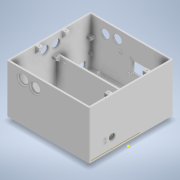
# Autodesk Inventor part: Base
Saved by Autodesk Inventor 2022.2 (Build 262287000, 287)
## iProperties
Created: 2022-01-15
Part Number: Base
Material: Generic
Document SubType Name: Modeling
Designer: siwat
Density: 1 g/cm^3
Appearance: Default
Mass: 201.568 g
Surface Area: 1377.7 cm^2
Volume: 201.568 cm^3
Author: siwat
Autodesk Inventor part; units mm, degrees
ref_plane "YZ Plane" through (0, 0, 0) normal (1, 0, 0) x (0, 1, 0)
ref_plane "XZ Plane" through (0, 0, 0) normal (0, 1, 0) x (-1, 0, 0)
ref_plane "XY Plane" through (0, 0, 0) normal (0, 0, 1) x (1, 0, 0)
ref_plane "Work Plane1" through (31.5112, 10.0003, 59.575) normal (-0.0015858, -0.9999987, 0.0000018) x (-0.0011293, 0, -0.9999994)
sketch "Sketch1" plane through (31.5112, 10.0003, 59.575) normal (-0.0015858, -0.9999987, 0.0000018) x (-0.0011293, 0, -0.9999994)
  line L0 (-4.5224, 4.5326) -> (134.4396, 4.5326)
  line L1 (134.4396, 4.5326) -> (134.4396, -131.8992)
  line L2 (134.4396, -131.8992) -> (-4.5224, -131.8992)
  line L3 (-4.5224, -131.8992) -> (-4.5224, 4.5326)
  line L4 (-7.5224, 7.5326) -> (137.4396, 7.5326)
  line L5 (137.4396, 7.5326) -> (137.4396, -134.8992)
  line L6 (137.4396, -134.8992) -> (-7.5224, -134.8992)
  line L7 (-7.5224, -134.8992) -> (-7.5224, 7.5326)
  point P0 (59.6106, -31.428)
  dimension "d0" = 138.9621
  dimension "d1" = 136.4319
  dimension "d2" = 74.8291
  dimension "d3" = 35.9607
  dimension "d4" = 3
  dimension "d5" = 3
  dimension "d6" = 3
  dimension "d7" = 3
  constraints: 16 end point, 4 parallel, 2 horizontal, 2 perpendicular
  measures "d0" distance between parallel lines of L1 L3
  measures "d1" distance between parallel lines of L0 L2
  measures "d2" distance from line of point (59.611, -31.428) L1
  measures "d3" distance from line of point (59.611, -31.428) L0
  measures "d4" distance between parallel lines of L0 L4
  measures "d5" distance between parallel lines of L3 L7
  measures "d6" distance between parallel lines of L5 L1
  measures "d7" distance between parallel lines of L6 L2
extrude "Extrusion1" add sketch "Sketch1" against normal blind 80
sketch "Sketch2" plane through (31.5112, 10.0003, 59.575) normal (-0.0015858, -0.9999987, 0.0000018) x (0.9999981, -0.0015858, -0.0011293)
  line L0 (-134.8992, -137.4396) -> (7.5326, -137.4396) projected
  line L1 (7.5326, 7.5224) -> (-134.8992, 7.5224) projected
  line L2 (7.5326, -137.4396) -> (-134.8992, -137.4396)
  line L3 (-134.8992, -137.4396) -> (-134.8992, 7.5224)
  line L4 (-134.8992, 7.5224) -> (7.5326, 7.5224)
  line L5 (7.5326, 7.5224) -> (7.5326, -137.4396)
  point P0 (-31.428, -59.6106)
  point P1 (-134.8992, -137.4396)
  point P2 (7.5326, 7.5224)
  constraints: 8 end point, 2 parallel, 1 horizontal, 1 perpendicular
extrude "Extrusion2" add sketch "Sketch2" along normal blind 3
sketch "Sketch3" plane through (31.5112, 10.0003, 59.575) normal (0.0015858, 0.9999987, -0.0000018) x (0.9999981, -0.0015858, -0.0011293)
  circle A0 centre (-112.8782, 129.2967) radius 1.9965
  circle A1 centre (-112.8782, 129.2967) radius 1
  circle A2 centre (-114.2274, 81.024) radius 1.9965
  circle A3 centre (-114.2274, 81.024) radius 1
  circle A4 centre (-62.1401, 86.0453) radius 1.9965
  circle A5 centre (-62.1401, 86.0453) radius 1
  circle A6 centre (-62.0938, 113.9832) radius 1.9965
  circle A7 centre (-62.0938, 113.9832) radius 1
  circle A8 centre (-37.9957, 129.2347) radius 1.9965
  circle A9 centre (-37.9957, 129.2347) radius 1
  circle A10 centre (-31.6312, 80.9446) radius 1.9965
  circle A11 centre (-31.6312, 80.9446) radius 1
  circle A12 centre (-6.6551, 121.5212) radius 2.3058
  circle A13 centre (-6.6551, 121.5212) radius 1
  circle A14 centre (-22.9352, 91.3493) radius 2.3058
  circle A15 centre (-22.9352, 91.3493) radius 1
  circle A16 centre (-129.08, 0.6108) radius 2.6932
  circle A17 centre (-129.08, 0.6108) radius 1
  circle A18 centre (-24.0772, 69.1234) radius 2.8442
  circle A19 centre (-24.0772, 69.1234) radius 1
  point P0 (-31.428, 59.6106)
  dimension "d12" = 2
  dimension "d13" = 2
  dimension "d14" = 2
  dimension "d15" = 2
  dimension "d16" = 2
  dimension "d17" = 2
  dimension "d18" = 2
  dimension "d19" = 2
  dimension "d28" = 2
  dimension "d29" = 2
  constraints: 20 centre point, 10 coincident
  measures "d12" diameter of A1
  measures "d13" diameter of A3
  measures "d14" diameter of A5
  measures "d15" diameter of A7
  measures "d16" diameter of A9
  measures "d17" diameter of A11
  measures "d18" diameter of A13
  measures "d19" diameter of A15
  measures "d28" diameter of A17
  measures "d29" diameter of A19
extrude "Extrusion3" add sketch "Sketch3" along normal blind 5
sketch "Sketch4" plane through (31.5112, 10.0003, 59.575) normal (0.0015858, 0.9999987, -0.0000018) x (0.9999981, -0.0015858, -0.0011293)
  line L0 (4.5326, 134.4396) -> (4.5326, -4.5224) projected
  line L1 (-131.8992, 134.4396) -> (-131.8992, -4.5224) projected
  line L2 (4.5326, 74.8611) -> (-131.8992, 74.8611)
  line L3 (-131.8992, 74.8611) -> (-131.8992, 77.8611)
  line L4 (-131.8992, 77.8611) -> (4.5326, 77.8611)
  line L5 (4.5326, 77.8611) -> (4.5326, 74.8611)
  point P0 (-31.428, 59.6106)
  point P1 (4.5326, 77.8611)
  point P2 (-131.8992, 74.8611)
  dimension "d22" = 3
  constraints: 8 end point, 2 parallel, 2 point on line, 1 horizontal, 1 perpendicular
  measures "d22" distance between parallel lines of L4 L2
extrude "Extrusion4" add sketch "Sketch4" along normal blind 50
sketch "Sketch5" plane through (35.9559, 9.9931, -18.2911) normal (-0.0011293, 0, -0.9999994) x (-0.9999981, 0.0015858, 0.0011293)
  circle A0 centre (12.779, 19.6609) radius 10
  point P0 (35.9607, -10.0501)
  dimension "d25" = 20
  constraints: 1 centre point
  measures "d25" diameter of A0
extrude "Extrusion5" cut sketch "Sketch5" against normal up to surface (3 mm away)
sketch "Sketch7" plane through (-100.5396, 10.2094, -74.7156) normal (0.9999981, -0.0015858, -0.0011293) x (-0.0011293, 0, -0.9999994)
  line L0 (0, 0) -> (0, 80) projected
  line L1 (0, 24.9377) -> (-4, 24.9377)
  line L2 (-4, 24.9377) -> (-4, 20.9377)
  line L3 (-4, 20.9377) -> (0, 20.9377)
  line L4 (0, 20.9377) -> (0, 24.9377)
  line L5 (-4, 24.9377) -> (-56.5786, 24.9377)
  line L6 (-56.5786, 50) -> (-56.5786, 0) projected
  line L7 (-4, 20.9377) -> (-56.5786, 20.9377)
  line L8 (-52.5786, 24.9377) -> (-52.5786, 20.9377)
  line L9 (-56.5786, 0) -> (-56.5786, 50) projected
  point P0 (-74.8291, -10.0501)
  point P1 (-56.5786, 90)
  dimension "d30" = 4
  dimension "d31" = 4
  dimension "d34" = 4
  constraints: 15 end point, 4 point on line, 3 horizontal, 2 parallel, 2 perpendicular
  measures "d30" distance of L3.end L2.end
  measures "d31" distance of L2.end L1.end
  measures "d34" distance from line of L6.start L8
extrude "Extrusion6" add sketch "Sketch7" along normal blind 4 contours L3 L2 L1 L0
sketch "Sketch8" plane through (-100.4955, 35.1471, -70.7156) normal (0.0015858, 0.9999987, -0.0000018) x (0.9999981, -0.0015858, -0.0011293)
  line L0 (136.4319, 4) -> (136.4319, -134.9621) projected
  line L1 (136.4319, 4) -> (129.4319, 4)
  line L2 (129.4319, 4) -> (129.4319, -3)
  line L3 (129.4319, -3) -> (136.4319, -3)
  line L4 (136.4319, -3) -> (136.4319, 4)
  line L5 (136.4319, -52.5786) -> (132.4319, -52.5786)
  line L6 (132.4319, -52.5786) -> (132.4319, -48.5786)
  line L7 (132.4319, -48.5786) -> (136.4319, -48.5786)
  line L8 (136.4319, -48.5786) -> (136.4319, -52.5786)
  line L9 (136.4319, 4) -> (0, 4) projected
  line L10 (0, -52.5786) -> (136.4319, -52.5786) projected
  line L11 (60.4128, -52.5786) -> (67.4128, -52.5786)
  line L12 (67.4128, -52.5786) -> (67.4128, -45.5786)
  line L13 (67.4128, -45.5786) -> (60.4128, -45.5786)
  line L14 (60.4128, -45.5786) -> (60.4128, -52.5786)
  circle A0 centre (132.9319, 0.5) radius 1.25
  circle A1 centre (63.9128, -49.0786) radius 1.25
  line L15 (0, -52.5786) -> (7, -52.5786)
  line L16 (7, -52.5786) -> (7, -45.5786)
  line L17 (7, -45.5786) -> (0, -45.5786)
  line L18 (0, -45.5786) -> (0, -52.5786)
  circle A2 centre (3.5, -49.0786) radius 1.25
  line L19 (64.4128, 4) -> (67.4128, 4)
  line L20 (67.4128, 4) -> (67.4128, 3)
  line L21 (67.4128, 3) -> (64.4128, 3)
  line L22 (64.4128, 3) -> (64.4128, 4)
  point P0 (100.4712, -70.8291)
  point P1 (67.4128, -52.5786)
  point P2 (7, -52.5786)
  point P3 (67.4128, 4)
  point P4 (64.4128, 4)
  dimension "d35" = 7
  dimension "d36" = 7
  dimension "d37" = 4
  dimension "d38" = 4
  dimension "d41" = 7
  dimension "d42" = 7
  dimension "d45" = 2.5
  dimension "d46" = 3.5
  dimension "d47" = 3.5
  dimension "d48" = 2.5
  dimension "d49" = 3.5
  dimension "d50" = 3.5
  dimension "d158" = 7
  dimension "d159" = 7
  dimension "d160" = 2.5
  dimension "d162" = 3
  dimension "d163" = 1
  dimension "d164" = 0
  dimension "d165" = 0
  dimension "d166" = 53.4128
  constraints: 40 end point, 10 parallel, 5 horizontal, 5 perpendicular, 3 centre point, 1 point on line
  measures "d35" distance of L3.end L2.end
  measures "d36" distance of L2.end L1.end
  measures "d37" distance of L6.end L7.end
  measures "d38" distance of L5.end L6.end
  measures "d41" distance of L13.end L12.end
  measures "d42" distance of L12.end L11.end
  measures "d45" diameter of A0
  measures "d46" distance from line of L9 A0.centre
  measures "d47" distance from line of L0 A0.centre
  measures "d48" diameter of A1
  measures "d49" distance from line of A1.centre L13
  measures "d50" distance from line of L12 A1.centre
  measures "d158" distance of L17.end L16.end
  measures "d159" distance of L16.end L15.end
  measures "d160" diameter of A2
  measures "d162" distance of L20.end L21.end
  measures "d163" distance of L19.end L20.end
  measures "d164" distance between parallel lines of L9 L19
  measures "d165" distance from line of L12 L19.end
  measures "d166" distance between parallel lines of L14 L16
extrude "Extrusion7" add sketch "Sketch8" against normal blind 4 contours L20 L21 L22 L9 | L18 L17 L16 L10 | L14 L13 L12 L10
sketch "Sketch11" plane through (31.5905, 60.0002, 59.5749) normal (0.0015858, 0.9999987, -0.0000018) x (0.9999981, -0.0015858, -0.0011293)
  line L0 (-131.8992, 74.8611) -> (-131.8992, 77.8611) projected
  line L1 (-131.8992, 74.8611) -> (-124.8992, 74.8611)
  line L2 (-124.8992, 74.8611) -> (-124.8992, 67.8611)
  line L3 (-124.8992, 67.8611) -> (-131.8992, 67.8611)
  line L4 (-131.8992, 67.8611) -> (-131.8992, 74.8611)
  line L5 (-131.8992, -4.5224) -> (4.5326, -4.5224) projected
  line L6 (4.5326, -4.5224) -> (-2.4674, -4.5224)
  line L7 (-2.4674, -4.5224) -> (-2.4674, 2.4776)
  line L8 (-2.4674, 2.4776) -> (4.5326, 2.4776)
  line L9 (4.5326, 2.4776) -> (4.5326, -4.5224)
  circle A0 centre (1.0326, -1.0224) radius 1.25
  circle A1 centre (-128.3992, 71.3611) radius 1.25
  line L10 (-131.8992, -4.5224) -> (-128.8992, -4.5224)
  line L11 (-128.8992, -4.5224) -> (-128.8992, -1.5224)
  line L12 (-128.8992, -1.5224) -> (-131.8992, -1.5224)
  line L13 (-131.8992, -1.5224) -> (-131.8992, -4.5224)
  line L14 (-131.8992, 74.8611) -> (4.5326, 74.8611) projected
  line L15 (4.5326, 74.8611) -> (1.5326, 74.8611)
  line L16 (1.5326, 74.8611) -> (1.5326, 71.8611)
  line L17 (1.5326, 71.8611) -> (4.5326, 71.8611)
  line L18 (4.5326, 71.8611) -> (4.5326, 74.8611)
  line L19 (-82.1632, -4.5224) -> (-79.1632, -4.5224)
  line L20 (-79.1632, -4.5224) -> (-79.1632, -1.5224)
  line L21 (-79.1632, -1.5224) -> (-82.1632, -1.5224)
  line L22 (-82.1632, -1.5224) -> (-82.1632, -4.5224)
  line L23 (4.5326, 74.8611) -> (-131.8992, 74.8611) projected
  line L24 (-82.1632, 74.8611) -> (-79.1632, 74.8611)
  line L25 (-79.1632, 74.8611) -> (-79.1632, 71.8611)
  line L26 (-79.1632, 71.8611) -> (-82.1632, 71.8611)
  line L27 (-82.1632, 71.8611) -> (-82.1632, 74.8611)
  line L28 (-40.7381, -4.5224) -> (-37.7381, -4.5224)
  line L29 (-37.7381, -4.5224) -> (-37.7381, -1.5224)
  line L30 (-37.7381, -1.5224) -> (-40.7381, -1.5224)
  line L31 (-40.7381, -1.5224) -> (-40.7381, -4.5224)
  line L32 (-40.7381, 74.8611) -> (-37.7381, 74.8611)
  line L33 (-37.7381, 74.8611) -> (-37.7381, 71.8611)
  line L34 (-37.7381, 71.8611) -> (-40.7381, 71.8611)
  line L35 (-40.7381, 71.8611) -> (-40.7381, 74.8611)
  line L36 (4.5326, 77.8611) -> (4.5326, 134.4396) projected
  line L37 (-131.8992, 134.4396) -> (-131.8992, 77.8611) projected
  line L38 (-131.8992, 134.4396) -> (-124.8992, 134.4396)
  line L39 (-124.8992, 134.4396) -> (-124.8992, 127.4396)
  line L40 (-124.8992, 127.4396) -> (-131.8992, 127.4396)
  line L41 (-131.8992, 127.4396) -> (-131.8992, 134.4396)
  circle A2 centre (-128.3992, 130.9396) radius 1.25 projected
  line L42 (-131.8992, 134.4396) -> (4.5326, 134.4396) projected
  line L43 (-37.7381, 134.4396) -> (-40.7381, 134.4396)
  line L44 (-40.7381, 134.4396) -> (-40.7381, 131.4396)
  line L45 (-40.7381, 131.4396) -> (-37.7381, 131.4396)
  line L46 (-37.7381, 131.4396) -> (-37.7381, 134.4396)
  line L47 (-79.1632, 134.4396) -> (-82.1632, 134.4396)
  line L48 (-82.1632, 134.4396) -> (-82.1632, 133.4396)
  line L49 (-82.1632, 133.4396) -> (-79.1632, 133.4396)
  line L50 (-79.1632, 133.4396) -> (-79.1632, 134.4396)
  line L51 (4.5326, 134.4396) -> (4.5326, -4.5224) projected
  line L52 (4.5326, 106.1504) -> (1.5326, 106.1504)
  line L53 (1.5326, 106.1504) -> (1.5326, 103.1504)
  line L54 (1.5326, 103.1504) -> (4.5326, 103.1504)
  line L55 (4.5326, 103.1504) -> (4.5326, 106.1504)
  point P0 (-31.428, 59.6106)
  point P1 (1.5326, 74.8611)
  point P2 (-2.4674, -4.5224)
  point P3 (-128.8992, -4.5224)
  point P4 (-37.7381, 74.8611)
  point P5 (-40.7381, 74.8611)
  point P6 (-79.1632, 74.8611)
  point P7 (-82.1632, 74.8611)
  point P8 (-79.1632, -4.5224)
  point P9 (-37.7381, -4.5224)
  point P10 (-2.4674, 134.4396)
  point P11 (-131.8992, 127.4396)
  point P12 (-82.1632, 134.4396)
  point P13 (-40.7381, 134.4396)
  point P14 (4.5326, 103.1504)
  point P15 (4.5326, 106.1504)
  dimension "d60" = 7
  dimension "d61" = 7
  dimension "d62" = 7
  dimension "d63" = 7
  dimension "d64" = 2.5
  dimension "d65" = 2.5
  dimension "d66" = 3
  dimension "d67" = 3
  dimension "d68" = 3
  dimension "d69" = 3
  dimension "d72" = 3
  dimension "d73" = 3
  dimension "d74" = 3
  dimension "d75" = 3
  dimension "d76" = 3
  dimension "d77" = 3
  dimension "d78" = 3
  dimension "d79" = 3
  dimension "d111" = 7
  dimension "d112" = 7
  dimension "d114" = 3
  dimension "d115" = 3
  dimension "d116" = 3
  dimension "d117" = 1
  dimension "d118" = 3
  dimension "d119" = 3
  constraints: 96 end point, 24 parallel, 12 horizontal, 12 perpendicular, 9 point on line, 2 centre point
  measures "d60" distance of L2.end L3.end
  measures "d61" distance of L1.end L2.end
  measures "d62" distance of L7.end L8.end
  measures "d63" distance of L6.end L7.end
  measures "d64" diameter of A0
  measures "d65" diameter of A1
  measures "d66" distance of L12.end L11.end
  measures "d67" distance of L11.end L10.end
  measures "d68" distance of L17.end L16.end
  measures "d69" distance of L16.end L15.end
  measures "d72" distance of L21.end L20.end
  measures "d73" distance of L20.end L19.end
  measures "d74" distance of L25.end L26.end
  measures "d75" distance of L24.end L25.end
  measures "d76" distance of L30.end L29.end
  measures "d77" distance of L29.end L28.end
  measures "d78" distance of L33.end L34.end
  measures "d79" distance of L32.end L33.end
  measures "d111" distance of L39.end L40.end
  measures "d112" distance of L38.end L39.end
  measures "d114" distance of L45.end L44.end
  measures "d115" distance of L44.end L43.end
  measures "d116" distance of L49.end L48.end
  measures "d117" distance of L48.end L47.end
  measures "d118" distance of L54.end L53.end
  measures "d119" distance of L53.end L52.end
extrude "Extrusion10" add sketch "Sketch11" against normal blind 4 contours L1 L2 L3 L4 | L37 L38 L39 L40 | L42 L50 L49 L48 | L14 L18 L17 L16 | L54 L53 L52 L36 | L13 L12 L11 L5 | L7 L8 L9 L5
sketch "Sketch12" plane through (39.1792, 89.9882, 67.0888) normal (0.9999981, -0.0015858, -0.0011293) x (-0.0011293, 0, -0.9999994)
  circle A0 centre (38.9565, -62.4338) radius 5
  line L0 (24.8703, -58.9338) -> (28.5014, -58.9338)
  line L1 (28.5014, -58.9338) -> (28.5014, -60.4338)
  line L2 (28.5014, -60.4338) -> (24.8703, -60.4338)
  line L3 (24.8703, -60.4338) -> (24.8703, -58.9338)
  line L4 (24.8703, -64.4338) -> (28.5014, -64.4338)
  line L5 (28.5014, -64.4338) -> (28.5014, -65.9338)
  line L6 (28.5014, -65.9338) -> (24.8703, -65.9338)
  line L7 (24.8703, -65.9338) -> (24.8703, -64.4338)
  point P0 (67.133, -90.0501)
  dimension "d80" = 10
  dimension "d179" = 1.5
  dimension "d180" = 1.5
  dimension "d181" = 4
  dimension "d182" = 2
  constraints: 16 end point, 4 parallel, 2 collinear, 2 horizontal, 2 perpendicular, 1 centre point
  measures "d80" diameter of A0
  measures "d179" distance of L0.end L1.end
  measures "d180" distance of L4.end L5.end
  measures "d181" distance between parallel lines of L4 L2
  measures "d182" distance from line of L2 A0.centre
extrude "Extrusion11" cut sketch "Sketch12" against normal up to surface (3 mm away)
sketch "Sketch13" plane through (-103.4161, 90.2141, -77.7123) normal (-0.9999981, 0.0015858, 0.0011293) x (0.0011293, 0, 0.9999994)
  line L0 (12.035, -65.9644) -> (29.035, -65.9644)
  line L1 (29.035, -65.9644) -> (29.035, -75.9644)
  line L2 (29.035, -75.9644) -> (12.035, -75.9644)
  line L3 (12.035, -75.9644) -> (12.035, -65.9644)
  point P0 (77.8291, -90.0501)
  dimension "d83" = 17
  dimension "d84" = 10
  constraints: 8 end point, 2 parallel, 1 horizontal, 1 perpendicular
  measures "d83" distance of L1.end L2.end
  measures "d84" distance of L0.end L1.end
extrude "Extrusion12" cut sketch "Sketch13" against normal up to surface (3 mm away)
sketch "Sketch14" plane through (-103.2524, 90.2141, 67.2496) normal (0.0011293, 0, 0.9999994) x (0.9999981, -0.0015858, -0.0011293)
  circle A0 centre (28.207, -14.6263) radius 6.9
  circle A1 centre (49.0395, -17.1012) radius 6.9
  point P0 (103.4712, -90.0501)
  dimension "d87" = 13.8
  dimension "d88" = 13.8
  constraints: 2 centre point
  measures "d87" diameter of A0
  measures "d88" diameter of A1
extrude "Extrusion13" cut sketch "Sketch14" against normal up to surface (3 mm away)
sketch "Sketch15" plane through (-103.4161, 90.2141, -77.7123) normal (-0.9999981, 0.0015858, 0.0011293) x (0.0011293, 0, 0.9999994)
  circle A0 centre (62.8637, -14.7589) radius 7
  circle A1 centre (82.5934, -14.7589) radius 7
  point P0 (77.8291, -90.0501)
  dimension "d91" = 14
  dimension "d124" = 14
  constraints: 2 centre point
  measures "d91" diameter of A0
  measures "d124" diameter of A1
extrude "Extrusion14" cut sketch "Sketch15" against normal up to surface (3 mm away)
sketch "Sketch16" plane through (39.0155, 89.9882, -77.8732) normal (-0.0011293, 0, -0.9999994) x (-0.9999981, 0.0015858, 0.0011293)
  line L0 (67.1739, -33.2483) -> (8.5598, -33.2483)
  line L1 (8.5598, -33.2483) -> (8.5598, -52.2542)
  line L2 (8.5598, -52.2542) -> (67.1739, -52.2542)
  line L3 (67.1739, -52.2542) -> (67.1739, -33.2483)
  circle A0 centre (69.1739, -31.2483) radius 1.5
  circle A1 centre (69.1739, -54.2542) radius 1.5
  circle A2 centre (6.5598, -54.2542) radius 1.5
  circle A3 centre (6.5598, -31.2483) radius 1.5
  point P0 (38.9607, -90.0501)
  dimension "d96" = 3
  dimension "d97" = 3
  dimension "d98" = 3
  dimension "d99" = 3
  dimension "d100" = 2
  dimension "d101" = 2
  dimension "d102" = 2
  dimension "d103" = 2
  dimension "d104" = 2
  dimension "d105" = 2
  dimension "d106" = 2
  dimension "d107" = 2
  constraints: 8 end point, 4 centre point, 2 parallel, 1 horizontal, 1 perpendicular
  measures "d96" diameter of A0
  measures "d97" diameter of A1
  measures "d98" diameter of A2
  measures "d99" diameter of A3
  measures "d100" distance from line of A3.centre L0
  measures "d101" horizontal distance of L0.end A3.centre
  measures "d102" distance from line of A0.centre L0
  measures "d103" distance from line of L3 A0.centre
  measures "d104" distance from line of L3 A1.centre
  measures "d105" distance from line of L2 A1.centre
  measures "d106" distance from line of A2.centre L1
  measures "d107" distance from line of L2 A2.centre
extrude "Extrusion15" cut sketch "Sketch16" against normal up to surface (3 mm away)
sketch "Sketch17" plane through (39.0155, 89.9882, -77.8732) normal (-0.0011293, 0, -0.9999994) x (-0.9999981, 0.0015858, 0.0011293)
  circle A0 centre (113.8306, -17.4407) radius 6.9
  circle A1 centre (92.9719, -14.7061) radius 6.9
  point P0 (38.9607, -90.0501)
  dimension "d120" = 13.8
  dimension "d121" = 13.8
  constraints: 2 centre point
  measures "d120" diameter of A0
  measures "d121" diameter of A1
extrude "Extrusion16" cut sketch "Sketch17" against normal up to surface (3 mm away)
fillet "Fillet1" radius 2 4 edges at (-103.3182, 48.7141, 67.2497) (39.1134, 48.4883, 67.0889) (38.9497, 48.4883, -77.8731) (-103.4819, 48.7141, -77.7123)
sketch "Sketch18" plane through (31.6381, 90.0002, 59.5749) normal (0.0015858, 0.9999987, -0.0000018) x (0.9999981, -0.0015858, -0.0011293)
  line L0 (4.5326, 77.8611) -> (4.5326, 134.4396) projected
  line L1 (4.5326, 101.4396) -> (-2.4674, 101.4396)
  line L2 (-2.4674, 101.4396) -> (-2.4674, 94.4396)
  line L3 (-2.4674, 94.4396) -> (4.5326, 94.4396)
  line L4 (4.5326, 94.4396) -> (4.5326, 101.4396)
  line L5 (4.5326, -4.5224) -> (4.5326, 74.8611) projected
  line L6 (4.5326, 28.4776) -> (-2.4674, 28.4776)
  line L7 (-2.4674, 28.4776) -> (-2.4674, 35.4776)
  line L8 (-2.4674, 35.4776) -> (4.5326, 35.4776)
  line L9 (4.5326, 35.4776) -> (4.5326, 28.4776)
  line L10 (-131.8992, 134.4396) -> (-131.8992, 77.8611) projected
  line L11 (-131.8992, 91.4396) -> (-124.8992, 91.4396)
  line L12 (-124.8992, 91.4396) -> (-124.8992, 84.4396)
  line L13 (-124.8992, 84.4396) -> (-131.8992, 84.4396)
  line L14 (-131.8992, 84.4396) -> (-131.8992, 91.4396)
  line L15 (-131.8992, -4.5224) -> (-131.8992, 134.4396) projected
  line L16 (-131.8992, 45.4776) -> (-124.8992, 45.4776)
  line L17 (-124.8992, 45.4776) -> (-124.8992, 38.4776)
  line L18 (-124.8992, 38.4776) -> (-131.8992, 38.4776)
  line L19 (-131.8992, 38.4776) -> (-131.8992, 45.4776)
  line L20 (-131.8992, 134.4396) -> (4.5326, 134.4396) projected
  line L21 (4.5326, -4.5224) -> (-131.8992, -4.5224) projected
  circle A0 centre (1.0326, 97.9396) radius 1.25
  circle A1 centre (1.0326, 31.9776) radius 1.25
  circle A2 centre (-128.3992, 41.9776) radius 1.25
  circle A3 centre (-128.3992, 87.9396) radius 1.25
  point P0 (-31.428, 59.6106)
  point P1 (-128.3992, 38.4776)
  point P2 (1.0326, 101.4396)
  point P3 (-131.8992, 38.4776)
  point P4 (4.5326, 35.4776)
  point P5 (4.5326, 94.4396)
  dimension "d126" = 7
  dimension "d127" = 7
  dimension "d128" = 7
  dimension "d129" = 7
  dimension "d130" = 7
  dimension "d131" = 7
  dimension "d132" = 7
  dimension "d133" = 7
  dimension "d134" = 43
  dimension "d135" = 43
  dimension "d136" = 33
  dimension "d137" = 33
  dimension "d138" = 2.5
  dimension "d139" = 2.5
  dimension "d140" = 2.5
  dimension "d141" = 2.5
  constraints: 32 end point, 8 parallel, 4 centre point, 4 horizontal, 4 perpendicular, 4 point on line, 2 midpoint
  measures "d126" distance of L3.end L2.end
  measures "d127" distance of L2.end L1.end
  measures "d128" distance of L7.end L8.end
  measures "d129" distance of L6.end L7.end
  measures "d130" distance of L12.end L13.end
  measures "d131" distance of L11.end L12.end
  measures "d132" distance of L17.end L18.end
  measures "d133" distance of L16.end L17.end
  measures "d134" distance between parallel lines of L20 L11
  measures "d135" distance from line of L21 point (-128.399, 38.478)
  measures "d136" distance from line of L21 L6.end
  measures "d137" distance from line of L20 point (1.033, 101.44)
  measures "d138" diameter of A0
  measures "d139" diameter of A1
  measures "d140" diameter of A2
  measures "d141" diameter of A3
extrude "Extrusion17" add sketch "Sketch18" against normal blind 5
draft "FaceDraft1" angle 45 pull direction (0.9999981, -0.0015858, -0.0011293) faces at (-96.8696, 85.2039, 14.9954) (-96.9153, 85.2039, -25.4727) fixed edges at (-93.3162, 85.1982, 17.7384) (-93.3682, 85.1982, -28.2237)
draft "FaceDraft6" angle 45 pull direction (-0.9999981, 0.0015858, 0.0011293) faces at (32.6055, 84.9984, -35.619) fixed edges at (29.0522, 85.0041, -38.3619)
draft "FaceDraft7" angle 45 pull direction (-0.9999981, 0.0015858, 0.0011293) faces at (32.5733, 84.9986, 24.8493) fixed edges at (29.1267, 85.0041, 27.6001)
sketch "Sketch19" plane through (39.1769, 89.9882, 65.0888) normal (0.9999981, -0.0015858, -0.0011293) x (-0.0011293, 0, -0.9999994)
  point P0 (65.133, -90.0501)
draft "FaceDraft8" angle 30 pull direction (0.0011293, 0, 0.9999994) faces at (-96.9487, 56.2039, -14.388) fixed edges at (-96.8915, 56.2038, -8.1411)
draft "FaceDraft9" angle 25 pull direction (-0.0011293, 0, -0.9999994) faces at (-96.9936, 31.1417, -18.894) fixed edges at (-96.9504, 31.1416, -25.1411)
draft "FaceDraft10" angle 40 pull direction (0.0011293, 0, 0.9999994) faces at (-35.0929, 31.0434, -74.1228) fixed edges at (-34.5925, 31.0426, -73.7901)
sketch "Sketch20" plane through (-101.2524, 90.2109, 67.2474) normal (0.0011293, 0, 0.9999994) x (0.9999981, -0.0015858, -0.0011293)
  circle A0 centre (26.207, -14.6263) radius 6.9 projected
  circle A1 centre (26.207, -14.6263) radius 8.95
  circle A2 centre (47.0395, -17.1012) radius 6.9 projected
  circle A3 centre (47.0395, -17.1012) radius 8.95
  point P0 (101.4712, -90.0501)
  dimension "d168" = 17.9
  dimension "d169" = 17.9
  constraints: 2 centre point, 2 coincident
  measures "d168" diameter of A1
  measures "d169" diameter of A3
extrude "Extrusion18" cut sketch "Sketch20" against normal blind 1.9
sketch "Sketch21" plane through (37.0155, 89.9914, -77.8709) normal (-0.0011293, 0, -0.9999994) x (-0.9999981, 0.0015858, 0.0011293)
  circle A0 centre (90.9719, -14.7061) radius 6.9 projected
  circle A1 centre (90.9719, -14.7061) radius 8.95
  circle A2 centre (111.8306, -17.4407) radius 6.9 projected
  circle A3 centre (111.8306, -17.4407) radius 8.95
  point P0 (36.9607, -90.0501)
  dimension "d172" = 17.9
  dimension "d173" = 17.9
  constraints: 2 centre point, 2 coincident
  measures "d172" diameter of A1
  measures "d173" diameter of A3
extrude "Extrusion19" cut sketch "Sketch21" against normal blind 1.9 contours A1 | A2 | A3
sketch "Sketch22" plane through (35.9559, 9.9931, -18.2911) normal (-0.0011293, 0, -0.9999994) x (-0.9999981, 0.0015858, 0.0011293)
  circle A0 centre (122.4956, 44.7688) radius 2.5
  point P0 (35.9607, -10.0501)
  dimension "d176" = 5
  constraints: 1 centre point
  measures "d176" diameter of A0
extrude "Extrusion20" cut sketch "Sketch22" against normal up to surface (3 mm away)
equation "\"d5\" = d4"
equation "\"d6\" = d4"
equation "\"d7\" = d5"
equation "\"d46\" = 0.5 * d36"
equation "\"d47\" = 0.5 * d35"
equation "\"d49\" = 0.5 * d41"
equation "\"d50\" = 0.5 * d42"
body "Solid1" dims "d126" = 7, "d127" = 7, "d137" = 33
